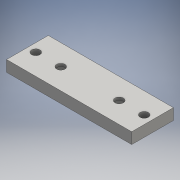
# Autodesk Inventor part: bearing support
Saved by Autodesk Inventor 2016 SP1 (Build 200210100, 210)
## iProperties
Created: 2016-05-25
Part Number: bearing support
Material: Generic
Document SubType Name: Modeling
Designer: ubik
Density: 1 g/cm^3
Appearance: Default
Author: ubik
Autodesk Inventor part; units mm, degrees
ref_plane "YZ Plane" through (0, 0, 0) normal (1, 0, 0) x (0, 1, 0)
ref_plane "XZ Plane" through (0, 0, 0) normal (0, 1, 0) x (-1, 0, 0)
ref_plane "XY Plane" through (0, 0, 0) normal (0, 0, 1) x (1, 0, 0)
sketch "Sketch1" plane through (0, 0, 0) normal (0, 0, 1) x (1, 0, 0)
  circle A0 centre (-21, 0) radius 8
  circle A1 centre (21, 0) radius 8
  line L0 (-45, 15) -> (45, 15)
  line L1 (45, 15) -> (45, -15)
  line L2 (45, -15) -> (-45, -15)
  line L3 (-45, -15) -> (-45, 15)
  point P0 (0, 0)
  dimension "d0" = 16
  dimension "d1" = 16
  dimension "d2" = 42
  dimension "d3" = 21
  dimension "d4" = 15
  dimension "d5" = 30
  dimension "d6" = 16
  dimension "d7" = 16
  constraints: 8 end point, 2 centre point, 2 parallel, 1 horizontal, 1 perpendicular
  measures "d0" diameter of A0
  measures "d1" diameter of A1
  measures "d2" distance of A1.centre A0.centre
  measures "d3" distance of point (0, 0) A0.centre
  measures "d4" distance from line of point (0, 0) L0
  measures "d5" distance of L2.end L0.start
  measures "d6" distance edge to line of A0 L3
  measures "d7" distance edge to line of A1 L1
extrude "Extrusion1" add sketch "Sketch1" along normal blind 8
sketch "Sketch2" plane through (0, 0, 8) normal (0, 0, 1) x (1, 0, 0)
  circle A0 centre (-21, 0) radius 8 projected
  circle A1 centre (21, 0) radius 8 projected
  point P0 (0, 0)
extrude "Extrusion2" add sketch "Sketch2" against normal blind 2
sketch "Sketch3" plane through (21, 0, 6) normal (0, 0, -1) x (-1, 0, 0)
  circle A0 centre (0, 0) radius 8 projected
  circle A1 centre (42, 0) radius 8 projected
  circle A2 centre (0, 0) radius 3
  circle A3 centre (42, 0) radius 3
  point P0 (21, 0)
  dimension "d12" = 6
  dimension "d13" = 6
  constraints: 2 centre point, 2 coincident
  measures "d12" diameter of A2
  measures "d13" diameter of A3
extrude "Extrusion3" cut sketch "Sketch3" against normal through all contours A2 | A3
sketch "Sketch4" plane through (0, 0, 8) normal (0, 0, 1) x (1, 0, 0)
  circle A0 centre (-39, 0) radius 3
  circle A1 centre (39, 0) radius 3
  line L0 (-45, 15) -> (-45, -15) projected
  line L1 (45, 15) -> (45, -15) projected
  point P0 (0, 0)
  dimension "d16" = 6
  dimension "d17" = 6
  dimension "d18" = 6
  dimension "d19" = 6
  constraints: 2 centre point
  measures "d16" diameter of A0
  measures "d17" diameter of A1
  measures "d18" distance from line of L0 A0.centre
  measures "d19" distance from line of L1 A1.centre
extrude "Extrusion4" cut sketch "Sketch4" against normal through all
equation "\"d1\" = d0"
equation "\"d3\" = 0.5 * d2"
equation "\"d4\" = 0.5 * d5"
equation "\"d7\" = d6"
equation "\"d19\" = d18"
body "Solid1"
